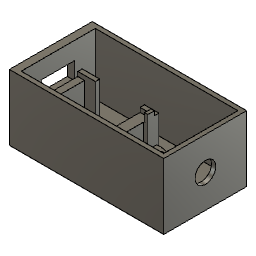
sustainpedaladapter (Autodesk Fusion 360 design; units mm, degrees)
Autodesk Fusion 360 part; units mm, degrees
note: some values were not read from the file. Chosen so that the rebuilt part matches the saved one: which bodies a step acts on; that a step has no effect; which face or edge a step refers to. Set by a fixed rule: which sketch regions a step uses.
mesh "Mesh1" [no effect]
sketch "Sketch1" plane through (0, 0, 0) normal (0, 1, 0) x (1, 0, 0)
  line L0 (5.974, 7.9901) -> (39.0126, 7.9901)
  line L1 (39.0126, 7.9901) -> (39.0126, -9.823)
  line L2 (39.0126, -9.823) -> (5.974, -9.823)
  line L3 (5.974, -9.823) -> (5.974, 7.9901)
  line L4 (5.974, 7.9901) -> (9.0811, 7.9901)
  line L5 (9.0811, 7.9901) -> (9.0811, -9.823)
  line L6 (9.0811, -9.823) -> (5.974, -9.823)
  line L7 (5.974, -9.823) -> (5.974, 7.9901)
  line L8 (39.0126, -9.823) -> (34.3859, -9.823)
  line L9 (34.3859, -9.823) -> (34.3859, 7.9901)
  line L10 (34.3859, 7.9901) -> (39.0126, 7.9901)
  line L11 (39.0126, 7.9901) -> (39.0126, -9.823)
  line L12 (5.974, -5.7061) -> (2.5758, -5.7061)
  line L13 (2.5758, -5.7061) -> (2.5758, 3.6442)
  line L14 (2.5758, 3.6442) -> (5.974, 3.6442)
  line L15 (5.974, 3.6442) -> (5.974, -5.7061)
  line L16 (5.974, -9.823) -> (6.2397, -9.823)
  line L17 (34.3859, 7.9901) -> (34.3859, 7.628)
  circle A0 centre (42.4562, -0.9165) radius 1.65
  line L18 (2.5758, -0.9165) -> (-6.804, -0.9165)
  line L19 (5.974, -5.7061) -> (9.0811, -5.7061)
  line L20 (5.974, 3.6442) -> (9.0811, 3.6442)
  line L21 (-5.3195, -19.823) -> (68.0159, -19.823)
  line L22 (-7.3968, 17.9901) -> (92.6032, 17.9901)
  line L23 (-8.6993, -17.823) -> (-6.9997, -17.823)
  line L24 (-6.9997, -17.823) -> (73.6693, -17.823)
  line L25 (-4.2299, 15.9901) -> (-3.0654, 15.9901)
  line L26 (-3.0654, 15.9901) -> (68.539, 15.9901)
  line L27 (71.0126, 17.9901) -> (71.0126, -22.0099)
  line L28 (73.0126, 24.8556) -> (73.0126, -24.6851)
  line L29 (68.0159, -19.823) -> (69.4863, -19.823)
  line L30 (69.4863, -19.823) -> (80.3336, -19.823)
  line L31 (68.539, 15.9901) -> (69.2143, 15.9901)
  line L32 (69.2143, 15.9901) -> (77.0897, 15.9901)
  line L33 (5.974, 7.9901) -> (5.974, 17.9901)
  line L34 (5.974, -9.823) -> (5.974, -19.823)
  line L35 (2.5758, 3.6442) -> (2.5758, 4.1982)
  line L36 (2.5758, 4.1982) -> (2.5758, 17.9901)
  line L37 (2.5758, -5.7061) -> (2.5758, -19.823)
  line L38 (45.9562, 1.1043) -> (42.4562, 3.125)
  line L39 (42.4562, 3.125) -> (38.9562, 1.1043)
  line L40 (38.9562, 1.1043) -> (38.9562, -2.9372)
  line L41 (38.9562, -2.9372) -> (42.4562, -4.9579)
  line L42 (42.4562, -4.9579) -> (45.9562, -2.9372)
  line L43 (45.9562, -2.9372) -> (45.9562, 1.1043)
  line L44 (39.0126, -0.9165) -> (40.8062, -0.9165)
  line L45 (44.1062, -0.9165) -> (76.6815, -0.9165)
  circle A1 centre (42.4562, -0.9165) radius 10
  circle A2 centre (42.4562, -0.9165) radius 3
  line L46 (39.0126, 7.9901) -> (41.0126, 7.9901)
  line L47 (41.0126, 7.9901) -> (41.0126, -9.823)
  line L48 (41.0126, -9.823) -> (39.0126, -9.823)
  line L49 (39.0126, -9.823) -> (39.0126, 7.9901)
  line L50 (39.0126, 4.9901) -> (41.0126, 4.9901)
  line L51 (39.0126, -6.823) -> (41.0126, -6.823)
  line L52 (41.0126, 7.9901) -> (34.3859, 7.9901)
  line L53 (34.3859, 7.9901) -> (34.3859, 9.9901)
  line L54 (34.3859, 9.9901) -> (41.0126, 9.9901)
  line L55 (41.0126, 9.9901) -> (41.0126, 7.9901)
  line L56 (34.3859, -9.823) -> (41.0126, -9.823)
  line L57 (41.0126, -9.823) -> (41.0126, -11.823)
  line L58 (41.0126, -11.823) -> (34.3859, -11.823)
  line L59 (34.3859, -11.823) -> (34.3859, -9.823)
  line L60 (5.974, -9.823) -> (13.974, -9.823)
  line L61 (13.974, -9.823) -> (13.974, -11.823)
  line L62 (13.974, -11.823) -> (5.974, -11.823)
  line L63 (5.974, -11.823) -> (5.974, -9.823)
  line L64 (5.974, 7.9901) -> (13.974, 7.9901)
  line L65 (13.974, 7.9901) -> (13.974, 9.9901)
  line L66 (13.974, 9.9901) -> (5.974, 9.9901)
  line L67 (5.974, 9.9901) -> (5.974, 7.9901)
  point P0 (42.4562, -0.9165)
  dimension "d7" = 3.3
  dimension "d18" = 10
  dimension "d19" = 10
  dimension "d20" = 8
  dimension "d21" = 8
  dimension "d22" = 100
  dimension "d23" = 32
  dimension "d24" = 40
  dimension "d25" = 2
  dimension "d47" = 3.5
  dimension "d48" = 20
  dimension "d55" = 6
  dimension "d70" = 2
  dimension "d71" = 3
  dimension "d72" = 3
  dimension "d87" = 2
  dimension "d88" = 2
  dimension "d89" = 8
  dimension "d90" = 2
  dimension "d91" = 8
  dimension "d92" = 2
  constraint horizontal L0
  constraint vertical L1
  constraint horizontal L2
  constraint vertical L3
  constraint horizontal L4
  constraint vertical L5
  constraint horizontal L6
  constraint vertical L7
  constraint coincident L2 L5.end
  constraint horizontal L8
  constraint vertical L9
  constraint horizontal L10
  constraint vertical L11
  constraint coincident L0 L9.end
  constraint horizontal L12
  constraint vertical L13
  constraint horizontal L14
  constraint vertical L15
  constraint coincident L7 L12.start
  constraint coincident L6 L16.end
  constraint coincident L9 L17.end
  constraint horizontal L44
  constraint coincident P0 L44
  constraint coincident L13 L18.start
  constraint coincident L1 L44.start
  constraint coincident L5 L19.end
  constraint perpendicular L5 L19
  constraint perpendicular L3 L20
  constraint horizontal L21
  constraint horizontal L22
  constraint parallel L2 L23
  constraint parallel L2 L24
  constraint parallel L22 L25
  constraint parallel L22 L26
  constraint coincident L22 L27.start
  constraint perpendicular L22 L27
  constraint vertical L28
  constraint parallel L21 L30
  constraint parallel L26 L32
  constraint coincident L22 L33.end
  constraint perpendicular L22 L33
  constraint coincident L21 L34.end
  constraint perpendicular L21 L34
  constraint coincident L22 L36.end
  constraint perpendicular L22 L36
  constraint coincident L21 L37.end
  constraint perpendicular L21 L37
  constraint coincident P0 A0.centre
  constraint coincident A0 L44.end
  constraint coincident A0 L45.start
  constraint collinear L44 L45
  constraint concentric A0 A1
  constraint concentric A0 A2
  constraint horizontal L46
  constraint vertical L47
  constraint horizontal L48
  constraint vertical L49
  constraint coincident L11 L50.start
  constraint coincident L47 L50.end
  constraint perpendicular L47 L50
  constraint coincident L49 L51.start
  constraint coincident L47 L51.end
  constraint perpendicular L47 L51
  constraint horizontal L52
  constraint vertical L53
  constraint horizontal L54
  constraint vertical L55
  constraint horizontal L56
  constraint vertical L57
  constraint horizontal L58
  constraint vertical L59
  constraint horizontal L60
  constraint vertical L61
  constraint horizontal L62
  constraint vertical L63
  constraint horizontal L64
  constraint vertical L65
  constraint horizontal L66
  constraint vertical L67
  measures "d7" diameter of A0
  measures "d18" distance of L2 L21
  measures "d19" distance of L0 L22
  measures "d20" distance of L2 L24
  measures "d21" distance of L0 L26
  measures "d22" distance of L22.start L22.end
  measures "d23" distance of L11 L27
  measures "d24" distance of L27.start L27.end
  measures "d25" distance of L27 L28
  measures "d47" distance of P0 L43
  measures "d48" diameter of A1
  measures "d55" diameter of A2
  measures "d70" distance of L0.end L46.end
  measures "d71" distance of L46 L50
  measures "d72" distance of L48 L51
  measures "d87" distance of L46.end L54.end
  measures "d88" distance of L8.end L58.end
  measures "d89" distance of L2.end L60.end
  measures "d90" distance of L2.end L62.end
  measures "d91" distance of L0.start L64.end
  measures "d92" distance of L0.start L66.end
extrude "Extrude7" add sketch "Sketch1" along normal blind 15 contours L22 L27 L28 L32 | L27 L28 L32 L45 | L24 L27 L28 L45 makes body 1
extrude "Extrude5" add sketch "Sketch1" against normal blind 3 separate body contours L0 L3 L4 L5 L7 L20 L64 | L3 L5 L7 L15 L19 L20 | L2 L3 L5 L6 L7 L16 L19 L60 | L0 L9 L10 L17 A1 L52 | L0 L1 L2 L8 L9 L10 L11 L39 L40 L41 A1 L49 L52 L56 | L2 L8 L9 A1 L56 | L1 L11 L39 L40 L41 L49 makes body 2 at (7.0097, 0, -2.0524) makes body 3 at (35.9281, 0, 3.8853)
extrude "Extrude3" add sketch "Sketch1" along normal blind 20 separate body contours A0 L47 | A0 L47 makes body 4
sketch "Sketch2" plane through (0, 0, 0) normal (1, 0, 0) x (0, 0, -1)
  circle A0 centre (0, 0) radius 4.75
  circle A1 centre (0, 0) radius 13
  dimension "d1" = 9.5
  dimension "d4" = 26
  constraint coincident A0.centre A1.centre
  constraint concentric A0 A1
  measures "d1" diameter of A0
  measures "d4" diameter of A1
extrude "Extrude1" add sketch "Sketch2" along normal blind 7 separate body contours A0 makes body 5
extrude "Extrude2" add sketch "Sketch2" against normal blind 26 separate body contours A0 | A1 makes body 6
combine "Combine1" operation add target body 5 tool bodies 6
extrude "Extrude4" add 1 faces at (41.8926, 0, 0.6124) along direction (0, -1, 0) blind 20 on bodies 4 bodies 4
move_body "Move1" bodies 5 to x (1, 0, 0) y (0, 1, 0) z (0, 0, 1) at (70.4684, 0, 0.796)
sketch "Sketch3" plane through (0, 0, 9.823) normal (0, 0, 1) x (1, 0, 0)
  line L0 (9.0811, 0) -> (5.974, 0)
  line L1 (5.974, 0) -> (5.974, -3)
  line L2 (5.974, -3) -> (9.0811, -3)
  line L3 (9.0811, -3) -> (9.0811, 0)
move_body "Move2" bodies 3 2 to x (1, 0, 0) y (0, 1, 0) z (0, 0, 1) at (0, 5, 0)
extrude "Extrude6" add sketch "Sketch1" against normal blind 3 separate body contours L0 L3 L4 L5 L7 L20 L64 | L3 L5 L7 L15 L19 L20 | L2 L3 L5 L6 L7 L16 L19 L60 | L0 L9 L10 L17 A1 L52 | L0 L1 L2 L8 L9 L10 L11 L39 L40 L41 A1 L49 L52 L56 | L2 L8 L9 A1 L56 | L1 L11 L39 L40 L41 L49 makes body 7 at (35.9281, 0, 3.8853) makes body 8 at (7.0097, 0, -2.0524)
copy_body "CutPasteBodies1" bodies 2 removing the originals makes body 9 in component "box"
copy_body "CutPasteBodies2" bodies 3 removing the originals makes body 10 in component "box"
copy_body "CutPasteBodies3" bodies 7 removing the originals makes body 11 in component "box"
copy_body "CutPasteBodies4" bodies 8 removing the originals makes body 12 in component "box"
extrude "Extrude1'" cut sketch "Sketch1" along normal blind 10 contours L3 L5 L7 L15 L19 L20 bodies 9 makes body 13 at (7.0097, 5, -6.5414) in component "box"
sketch "Sketch4" plane through (0, 0, 0) normal (0, 1, 0) x (1, 0, 0)
copy_body "CutPasteBodies5" bodies 1 removing the originals makes body 14 in component "box"
extrude "Extrude3'" add sketch "Sketch1" along normal blind 15 separate body contours L3 L7 L14 L26 L33 L35 L36 L67 | L3 L7 L12 L13 L14 L15 | L3 L7 L12 L24 L34 L37 L63 | L22 L26 L27 L31 L32 L33 | L22 L26 L33 L36 | L21 L24 L34 L37 | L21 L24 L27 L29 L30 L34 | L24 L27 L28 L30 makes body 15 in component "box"
extrude "Extrude4'" cut sketch "Sketch1" along normal blind 5 contours L3 L7 L12 L13 L14 L15 bodies 9 10 11 12 13 14 15 in component "box"
extrude "Extrude5'" add sketch "Sketch1" along normal blind 2 separate body contours L0 L4 L33 L64 L65 L66 L67 | L0 L3 L4 L5 L7 L20 L64 | L0 L2 L5 L9 L17 A1 L60 L64 | L3 L5 L7 L15 L19 L20 | L0 L26 L27 L31 L32 L33 L45 A1 L53 L54 L55 L65 L66 | L2 L3 L5 L6 L7 L16 L19 L60 | L0 L10 A1 L52 L53 L54 L55 | L0 L9 L10 L17 A1 L52 | L2 L6 L16 L34 L60 L61 L62 L63 | L0 L10 A1 L46 L52 L55 | L0 L1 L2 L8 L9 L10 L11 L39 L40 L41 A1 L49 L52 L56 | L2 L24 L27 L34 L45 A1 L57 L58 L59 L61 L62 | L1 L11 L46 L47 L49 L50 L52 | L38 L39 L43 L45 A1 L47 L55 | L9 A1 | L1 L11 L39 L47 L49 L50 | L41 L42 L43 L45 A1 L47 L57 | L2 L8 L9 A1 L56 | L2 L8 A1 L56 L57 L58 L59 | L1 L11 L39 L44 A2 L47 L49 | L1 L11 L39 L40 L41 L49 | L38 L39 L43 L45 A2 L47 | L41 L42 L43 L45 A2 L47 | L2 L8 A1 L48 L56 L57 | L1 L11 L41 L44 A2 L47 L49 | A0 L45 A2 L47 | A0 L45 A2 L47 | L1 L11 L47 L48 L49 L51 L56 | L1 L11 L41 L47 L49 L51 | A0 L44 A2 L47 | A0 L44 A2 L47 | A0 L47 | A0 L47 makes body 16 in component "box"
move_body "Move1'" bodies 16 to x (1, 0, 0) y (0, 1, 0) z (0, 0, 1) at (0, 13, 0) in component "box"
extrude "Extrude8" add 2 faces at (7.0097, 5, 7.0784) (7.0097, 5, -6.5414) along direction (0, 1, 0) blind 10 separate body on bodies 9 13 makes body 17 at (5.974, 8.3333, 8.4507) makes body 18 at (9.0811, 8.3333, -6.5414)
extrude "Extrude6'" add 1 faces at (35.9281, 5, 3.8853) along direction (0, 1, 0) blind 10 on bodies 10 bodies 10 in component "box"
combine "Combine1'" operation add target body 9 tool bodies 17 in component "box"
combine "Combine2" operation add target body 18 tool bodies 13
combine "Combine2'" operation add target body 9 tool bodies 10 18 16 in component "box"
combine "Combine3" operation add target body 14 tool bodies 15 in component "box"
extrude "Extrude9" add sketch "Sketch1" against normal blind 15 separate body contours L3 L7 L14 L26 L33 L35 L36 L67 | L3 L7 L12 L13 L14 L15 | L3 L7 L12 L24 L34 L37 L63 | L22 L26 L27 L31 L32 L33 | L22 L26 L33 L36 | L21 L24 L34 L37 | L22 L27 L28 L32 | L21 L24 L27 L29 L30 L34 | L27 L28 L32 L45 | L24 L27 L28 L45 | L24 L27 L28 L30 makes body 19
extrude "Extrude10" add sketch "Sketch1" against normal blind 2 separate body contours L0 L4 L33 L64 L65 L66 L67 | L0 L3 L4 L5 L7 L20 L64 | L0 L2 L5 L9 L17 A1 L60 L64 | L3 L5 L7 L15 L19 L20 | L0 L26 L27 L31 L32 L33 L45 A1 L53 L54 L55 L65 L66 | L2 L3 L5 L6 L7 L16 L19 L60 | L0 L10 A1 L52 L53 L54 L55 | L0 L9 L10 L17 A1 L52 | L2 L6 L16 L34 L60 L61 L62 L63 | L0 L10 A1 L46 L52 L55 | L0 L1 L2 L8 L9 L10 L11 L39 L40 L41 A1 L49 L52 L56 | L2 L24 L27 L34 L45 A1 L57 L58 L59 L61 L62 | L1 L11 L46 L47 L49 L50 L52 | L38 L39 L43 L45 A1 L47 L55 | L9 A1 | L1 L11 L39 L47 L49 L50 | L41 L42 L43 L45 A1 L47 L57 | L2 L8 L9 A1 L56 | L2 L8 A1 L56 L57 L58 L59 | L1 L11 L39 L44 A2 L47 L49 | L1 L11 L39 L40 L41 L49 | L38 L39 L43 L45 A2 L47 | L41 L42 L43 L45 A2 L47 | L2 L8 A1 L48 L56 L57 | L1 L11 L41 L44 A2 L47 L49 | A0 L45 A2 L47 | A0 L45 A2 L47 | L1 L11 L47 L48 L49 L51 L56 | L1 L11 L41 L47 L49 L51 | A0 L44 A2 L47 | A0 L44 A2 L47 | A0 L47 | A0 L47 makes body 20
move_body "Move3" bodies 20 to x (1, 0, 0) y (0, 1, 0) z (0, 0, 1) at (0, -13, 0)
extrude "Extrude7'" add 2 faces at (7.0097, -3, -2.0524) (35.9281, -3, 3.8853) along direction (0, -1, 0) blind 11 on bodies 11 12 bodies 12 11 in component "box"
combine "Combine3'" operation add target body 20 tool bodies 19
combine "Combine4" operation add target body 20 tool bodies 12
combine "Combine4'" operation add target body 11 tool bodies 20 in component "box"
combine "Combine5" operation add target body 11 tool bodies 14 in component "box"
combine "Combine6" operation cut target body 11 tool bodies 4 in component "box"
sketch "Sketch5" plane through (0, -15, 0) normal (0, -1, 0) x (1, 0, 0)
  circle A0 centre (42.4562, 0.9165) radius 1.65
  line L0 (2.5758, 19.823) -> (2.5758, -17.9901)
  line L1 (2.5758, -17.9901) -> (73.0126, -17.9901)
  line L2 (73.0126, -17.9901) -> (73.0126, 19.823)
  line L3 (73.0126, 19.823) -> (2.5758, 19.823)
  circle A1 centre (42.4562, 0.9165) radius 1.5
  dimension "d46" = 3
  constraint concentric A0 A1
  measures "d46" diameter of A1
extrude "Extrude11" add sketch "Sketch1" along normal blind 5 separate body contours L0 L10 A1 L46 L52 L55 | L0 L1 L2 L8 L9 L10 L11 L39 L40 L41 A1 L49 L52 L56 | L1 L11 L46 L47 L49 L50 L52 | L38 L39 L43 L45 A1 L47 L55 | L9 A1 | L1 L11 L39 L47 L49 L50 | L41 L42 L43 L45 A1 L47 L57 | L1 L11 L39 L44 A2 L47 L49 | L1 L11 L39 L40 L41 L49 | L38 L39 L43 L45 A2 L47 | L41 L42 L43 L45 A2 L47 | L2 L8 A1 L48 L56 L57 | L1 L11 L41 L44 A2 L47 L49 | A0 L45 A2 L47 | A0 L45 A2 L47 | L1 L11 L47 L48 L49 L51 L56 | L1 L11 L41 L47 L49 L51 | A0 L44 A2 L47 | A0 L44 A2 L47 makes body 21
move_body "Move4" bodies 21 to x (1, 0, 0) y (0, 1, 0) z (0, 0, 1) at (0, -15, 0)
combine "Combine7" operation add target body 11 tool bodies 21 in component "box"
extrude "Extrude12" add sketch "Sketch1" along normal blind 2 separate body contours L1 L11 L39 L44 A2 L47 L49 | L1 L11 L39 L40 L41 L49 | L38 L39 L43 L45 A2 L47 | L41 L42 L43 L45 A2 L47 | L1 L11 L41 L44 A2 L47 L49 | A0 L45 A2 L47 | A0 L45 A2 L47 | A0 L44 A2 L47 | A0 L44 A2 L47 | A0 L47 | A0 L47 makes body 22
move_body "Move5" bodies 22 to x (1, 0, 0) y (0, 1, 0) z (0, 0, 1) at (0, -15, 0)
combine "Combine8" operation cut target body 11 tool bodies 22 in component "box"
combine "Combine9" operation cut target body 11 tool bodies 5 keep tools in component "box"
extrude "Extrude13" add sketch "Sketch1" along normal blind 2 separate body contours L0 L10 A1 L46 L52 L55 | L0 L1 L2 L8 L9 L10 L11 L39 L40 L41 A1 L49 L52 L56 | L1 L11 L46 L47 L49 L50 L52 | L38 L39 L43 L45 A1 L47 L55 | L9 A1 | L1 L11 L39 L47 L49 L50 | L41 L42 L43 L45 A1 L47 L57 | L1 L11 L39 L44 A2 L47 L49 | L1 L11 L39 L40 L41 L49 | L38 L39 L43 L45 A2 L47 | L41 L42 L43 L45 A2 L47 | L2 L8 A1 L48 L56 L57 | L1 L11 L41 L44 A2 L47 L49 | A0 L45 A2 L47 | A0 L45 A2 L47 | L1 L11 L47 L48 L49 L51 L56 | L1 L11 L41 L47 L49 L51 | A0 L44 A2 L47 | A0 L44 A2 L47 | A0 L47 | A0 L47 makes body 23
move_body "Move6" bodies 23 to x (1, 0, 0) y (0, 1, 0) z (0, 0, 1) at (0, 11, 0)
extrude "Extrude14" add sketch "Sketch1" along normal blind 2 separate body contours A0 L45 A2 L47 | A0 L45 A2 L47 | A0 L44 A2 L47 | A0 L44 A2 L47 | A0 L47 | A0 L47 makes body 24
move_body "Move7" bodies 24 to x (1, 0, 0) y (0, 1, 0) z (0, 0, 1) at (0, 13, 0)
combine "Combine10" operation cut target body 9 tool bodies 24 in component "box"
combine "Combine11" operation add target body 9 tool bodies 23 in component "box"
extrude "Extrude8'" cut sketch "Sketch1" along normal blind 34 contours A0 L47 | A0 L47 bodies 9 in component "box"
extrude "Extrude9'" cut 1 faces at (71.0126, 13.6667, -4.7191) along direction (-1, 0, 0) blind 0.3 on bodies 9 bodies 9 in component "box"
extrude "Extrude10'" cut 1 faces at (27.5535, 13.6667, -15.9901) along direction (0, 0, 1) blind 0.3 on bodies 9 bodies 9 in component "box"
extrude "Extrude11'" cut 1 faces at (5.974, 5.6667, -6.5414) along direction (1, 0, 0) blind 0.3 on bodies 9 bodies 9 in component "box"
extrude "Extrude12'" cut 1 faces at (27.7535, 13.6667, 17.823) along direction (0, 0, -1) blind 0.3 on bodies 9 bodies 9 in component "box"
combine "Combine12" operation cut target body 9 tool bodies 5 keep tools in component "box"
extrude "Extrude13'" cut 1 faces at (43.8978, -13, 3.4135) along direction (0, 1, 0) blind 0.5 on bodies 11 bodies 11 in component "box"
extrude "Extrude14'" add sketch "Sketch1" against normal blind 12 contours L1 L11 L46 L47 L49 L50 L52 | L1 L11 L47 L48 L49 L51 L56 bodies 11 in component "box"
extrude "Extrude15" add sketch "Sketch1" along normal blind 4 contours L1 L11 L46 L47 L49 L50 L52 | L1 L11 L47 L48 L49 L51 L56 bodies 11 in component "box"
extrude "Extrude16" cut 2 faces at (39.0126, 1.3333, -6.9901) (39.0126, 1.3333, 7.823) along direction (1, 0, 0) blind 0.5 on bodies 11 bodies 11 in component "box"
extrude "Extrude17" cut 1 faces at (3.7086, 1.6667, -3.6442) along direction (0, 0, -1) blind 3 on bodies 11 bodies 11 in component "box"
extrude "Extrude18" cut 1 faces at (4.8413, 1.6667, 5.7061) along direction (0, 0, 1) blind 3 on bodies 11 bodies 11 in component "box"
extrude "Extrude19" cut 1 faces at (3.7086, 5, -1.5274) along direction (0, 1, 0) blind 2 on bodies 11 bodies 11 in component "box"
sketch "Sketch6" plane through (0, 0, 0) normal (0, 1, 0) x (-1, 0, 0)
  line L0 (-5.974, 8.7061) -> (-5.974, 9.823)
  line L1 (-5.974, 9.823) -> (-9.0811, 9.823)
  line L2 (-9.0811, 9.823) -> (-9.0811, -7.9901)
  line L3 (-9.0811, -7.9901) -> (-5.974, -7.9901)
  line L4 (-5.974, -7.9901) -> (-5.974, -6.6442)
  line L5 (-5.974, -6.6442) -> (-2.5758, -6.6442)
  line L6 (-2.5758, -6.6442) -> (-2.5758, 8.7061)
  line L7 (-2.5758, 8.7061) -> (-5.974, 8.7061)
  line L8 (-5.974, -6.6442) -> (-5.974, -6.3762)
  line L9 (-5.974, -6.3762) -> (-5.974, 8.7061)
  constraint coincident L4.end L5.start
  constraint perpendicular L5 L8
  constraint coincident L0.start L7.end
extrude "Extrude20" cut sketch "Sketch6" against normal blind 1 contours L5 L6 L7 L8 L9 bodies 11 in component "box"
extrude "Extrude15'" add sketch "Sketch1" along normal blind 2 separate body contours L0 L4 L33 L64 L65 L66 L67 | L0 L10 A1 L52 L53 L54 L55 | L2 L6 L16 L34 L60 L61 L62 L63 | L0 L10 A1 L46 L52 L55 | L2 L8 A1 L56 L57 L58 L59 | L2 L8 A1 L48 L56 L57 makes body 25 at (8.6407, 0, -8.6567) makes body 26 at (38.8037, 0, 10.4896) makes body 27 at (8.6407, 0, 10.4896) makes body 28 at (36.5948, 0, -9.3234)
extrude "Extrude16'" add sketch "Sketch1" against normal blind 13 separate body contours L0 L4 L33 L64 L65 L66 L67 | L0 L10 A1 L52 L53 L54 L55 | L2 L6 L16 L34 L60 L61 L62 L63 | L0 L10 A1 L46 L52 L55 | L2 L8 A1 L56 L57 L58 L59 | L2 L8 A1 L48 L56 L57 makes body 29 at (38.8037, -4.3333, 9.823) makes body 30 at (36.5948, -4.3333, -7.9901) makes body 31 at (11.3073, -4.3333, 11.823) makes body 32 at (11.3073, -4.3333, -9.9901)
combine "Combine5'" operation add target body 25 tool bodies 26 27 28 30 31 29 32 keep tools makes body 33 at (11.3073, -8, 11.823) makes body 34 at (38.8037, -8, 9.823) makes body 35 at (38.8037, -3, -7.9901)
extrude "Extrude19'" cut 1 faces at (38.8037, 0.6667, 9.823) along direction (0, 0, 1) blind 0.5 on bodies 26 bodies 26 34
combine "Combine6'" operation add target body 25 tool bodies 26 27 28 35 34 33 32 29 30 31 11
component "box" placed x (1, 0, 0) y (0, 1, 0) z (0, 0, 1) at (0, 0, 0)
hidden bodies 5 9
named bodies: "jack", "drill", "top", "bottom"
